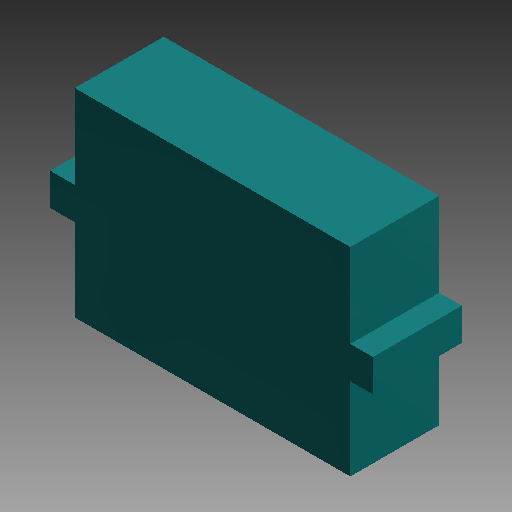
# Autodesk Inventor part: SZMM3Z4V7T1G
Saved by Autodesk Inventor 2018.2 (Build 222227000, 227)
## iProperties
Part Number: SZMM3Z4V7T1G
Material: Generic
Document SubType Name: Modeling
Designer: autocad
Appearance: SOD323-R, SZMM3Z4V7T1G
Author: autocad
Autodesk Inventor part; units mm, degrees
ref_plane "YZ Plane" through (0, 0, 0) normal (1, 0, 0) x (0, 1, 0)
ref_plane "XZ Plane" through (0, 0, 0) normal (0, 1, 0) x (-1, 0, 0)
ref_plane "XY Plane" through (0, 0, 0) normal (0, 0, 1) x (1, 0, 0)
sketch "SOD323-R, SZMM3Z4V7T1G_137" plane through (0, 0, 0) normal (0, 0, 1) x (1, 0, 0)
  line L0 (1.0922, -0.127) -> (1.0922, -0.7762)
  line L1 (1.0922, -0.7762) -> (-1.0762, -0.7762)
  line L2 (-1.0762, -0.7762) -> (-1.0762, -0.127)
  line L3 (-1.0762, -0.127) -> (-1.27, -0.127)
  line L4 (-1.27, -0.127) -> (-1.27, 0.127)
  line L5 (-1.27, 0.127) -> (-1.0762, 0.127)
  line L6 (-1.0762, 0.127) -> (-1.0762, 0.7874)
  line L7 (-1.0762, 0.7874) -> (1.0922, 0.7874)
  line L8 (1.0922, 0.7874) -> (1.0922, 0.127)
  line L9 (1.0922, 0.127) -> (1.27, 0.127)
  line L10 (1.27, 0.127) -> (1.27, -0.127)
  line L11 (1.27, -0.127) -> (1.0922, -0.127)
  constraints: 24 end point
extrude "Extrusion1" add sketch "SOD323-R, SZMM3Z4V7T1G_137" along normal blind 0.7
body "Solid1"
